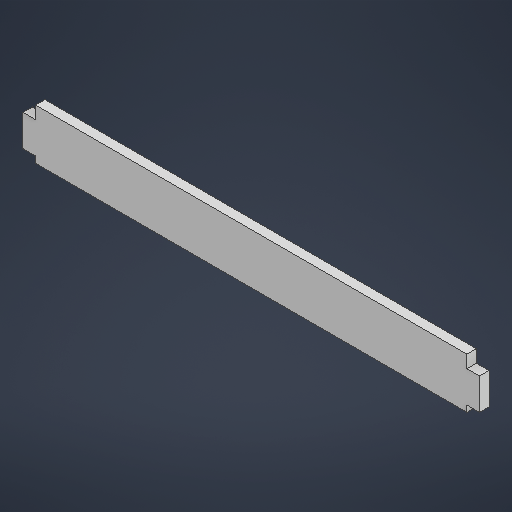
# Autodesk Inventor part: Battary_holder_part3
Saved by Autodesk Inventor 2027 (Build 310192000, 192)
## iProperties
Created: 2026-05-15
Part Number: Battary_holder_part3
Material: Generic
Document SubType Name: Modeling
Designer: alexy
Density: 1 g/cm^3
Appearance: Default
Author: alexy
Autodesk Inventor part; units mm, degrees
ref_plane "YZ Plane" through (0, 0, 0) normal (1, 0, 0) x (0, 1, 0)
ref_plane "XZ Plane" through (0, 0, 0) normal (0, 1, 0) x (-1, 0, 0)
ref_plane "XY Plane" through (0, 0, 0) normal (0, 0, 1) x (1, 0, 0)
sketch "Sketch1" plane through (0, 0, 0) normal (0, 0, 1) x (1, 0, 0)
  line L0 (0, 0) -> (137, 0)
  line L1 (137, 0) -> (137, 16)
  line L2 (137, 16) -> (0, 16)
  line L3 (0, 16) -> (0, 0)
  line L4 (-4, 12) -> (0, 12)
  line L5 (0, 12) -> (0, 2)
  line L6 (0, 2) -> (-4, 2)
  line L7 (-4, 2) -> (-4, 12)
  line L8 (-4, 12) -> (0, 2) construction
  line L9 (0, 12) -> (-4, 2) construction
  line L10 (141, 12) -> (137, 12)
  line L11 (137, 12) -> (137, 2)
  line L12 (137, 2) -> (141, 2)
  line L13 (141, 2) -> (141, 12)
  line L14 (141, 12) -> (137, 2) construction
  line L15 (137, 12) -> (141, 2) construction
  point P0 (-2, 7)
  point P1 (0, 8)
  point P2 (139, 7)
  point P3 (0, 12)
  dimension "d0" = 137
  dimension "d1" = 16
  dimension "d2" = 4
  dimension "d3" = 10
  dimension "d4" = 4
  dimension "d7" = 2
  constraints: 32 end point, 6 parallel, 5 midpoint, 3 horizontal, 3 perpendicular, 2 horizontal alignment, 2 point on line
  measures "d0" distance of L0.start L0.end
  measures "d1" distance of L0.end L1.end
  measures "d2" distance of L4.start L4.end
  measures "d3" distance of L6.end L4.start
  measures "d4" distance of L10.start L10.end
  measures "d7" distance from line of L0.start L6
extrude "Extrusion1" add sketch "Sketch1" along normal blind 3
body "Solid1"
